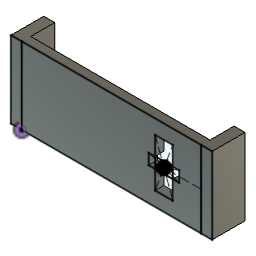
ClipHolder v4 (Autodesk Fusion 360 design; units mm, degrees)
Autodesk Fusion 360 part; units mm, degrees
sketch "Sketch1" plane through (0, 0, 0) normal (0, 1, 0) x (1, 0, 0)
  line L0 (0, 0) -> (82, 0)
  line L1 (82, 0) -> (82, -35)
  line L2 (82, -35) -> (0, -35)
  line L3 (0, -35) -> (0, 0)
  line L4 (82, -17.5) -> (69, -17.5) construction
  line L5 (69, -17.5) -> (64.95, -17.5) construction
  line L6 (60.9, -6.45) -> (69, -6.45)
  line L7 (69, -6.45) -> (69, -28.55)
  line L8 (69, -28.55) -> (60.9, -28.55)
  line L9 (60.9, -28.55) -> (60.9, -6.45)
  line L10 (60.9, -6.45) -> (69, -28.55) construction
  line L11 (69, -6.45) -> (60.9, -28.55) construction
  line L12 (82, -35) -> (87, -35)
  line L13 (87, -35) -> (87, 0)
  line L14 (87, 0) -> (82, 0)
  line L15 (82, 0) -> (82, -35)
  line L16 (0, -35) -> (-5, -35)
  line L17 (-5, -35) -> (-5, 0)
  line L18 (-5, 0) -> (0, 0)
  line L19 (0, 0) -> (0, -35)
  line L20 (71.95, -20) -> (57.95, -20)
  line L21 (57.95, -20) -> (57.95, -15)
  line L22 (57.95, -15) -> (71.95, -15)
  line L23 (71.95, -15) -> (71.95, -20)
  line L24 (71.95, -20) -> (57.95, -15) construction
  line L25 (57.95, -20) -> (71.95, -15) construction
  point P0 (64.95, -17.5)
  point P1 (64.95, -17.5)
  dimension "d1" = 82
  dimension "d2" = 35
  dimension "d3" = 13
  dimension "d4" = 4.05
  dimension "d5" = 8.1
  dimension "d6" = 22.1
  dimension "d7" = 5
  dimension "d8" = 35
  dimension "d9" = 5
  dimension "d10" = 35
  dimension "d15" = 14
  dimension "d16" = 5
  constraint horizontal L0
  constraint vertical L1
  constraint horizontal L2
  constraint vertical L3
  constraint coincident L0.start L3.end
  constraint midpoint L1 L4.start
  constraint perpendicular L1 L4
  constraint parallel L4 L5
  constraint horizontal L6
  constraint perpendicular L6 L7
  constraint parallel L6 L8
  constraint parallel L7 L9
  constraint coincident L10 P1
  constraint coincident L11 P1
  constraint coincident P1 P0
  constraint horizontal L12
  constraint vertical L13
  constraint horizontal L14
  constraint vertical L15
  constraint horizontal L16
  constraint vertical L17
  constraint horizontal L18
  constraint vertical L19
  constraint horizontal L20
  constraint perpendicular L20 L21
  constraint parallel L20 L22
  constraint parallel L21 L23
  constraint coincident L24 P1
  constraint coincident L25 P1
  measures "d1" distance of L0.start L0.end
  measures "d2" distance of L0.start L2.end
  measures "d3" distance of L4.start L4.end
  measures "d4" distance of L4.end P1
  measures "d5" distance of L7.end L8.end
  measures "d6" distance of L6.end L7.end
  measures "d7" distance of L1.end L12.end
  measures "d8" distance of L1.end L0.end
  measures "d9" distance of L2.end L16.end
  measures "d10" distance of L2.end L0.start
  measures "d15" distance of L21.end L22.end
  measures "d16" distance of L20.end L21.end
extrude "Extrude1" add sketch "Sketch1" along normal blind 15 contours L3 L16 L17 L18 L19 | L1 L12 L13 L14 L15 makes body 1 at (0, 5, 23.3333) makes body 2 at (87, 5, 23.3333)
extrude "Extrude2" add sketch "Sketch1" along normal blind 4 contours L0 L1 L2 L3 L15 L19 | L9 L20 L21 L22 | L7 L20 L22 L23 bodies 1 2
extrude "Extrude3" cut sketch "Sketch1" along normal blind 4 contours L9 L20 L21 L22 | L7 L20 L22 L23 bodies 1
equation "d4 = ( 8.1 / 2 ) * 1 mm"
